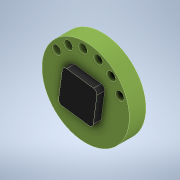
# Autodesk Inventor part: FootSensorPCB
Saved by Autodesk Inventor 2022 (Build 260153000, 153)
## iProperties
Created: 2021-12-28
Part Number: FootSensorPCB
Material: Generic
Document SubType Name: Modeling
Designer: Jochen
Density: 1 g/cm^3
Appearance: Olive Green
Author: Jochen
Autodesk Inventor part; units mm, degrees
ref_plane "YZ Plane" through (0, 0, 0) normal (1, 0, 0) x (0, 1, 0)
ref_plane "XZ Plane" through (0, 0, 0) normal (0, 1, 0) x (-1, 0, 0)
ref_plane "XY Plane" through (0, 0, 0) normal (0, 0, 1) x (1, 0, 0)
sketch "Sketch1" plane through (0, 0, 0) normal (0, 0, 1) x (1, 0, 0)
  line L0 (0, -7) -> (0, 7) construction
  line L1 (-7, 0) -> (7, 0) construction
  circle A0 centre (0, 0) radius 5
  circle A1 centre (0, 0) radius 4.2 construction
  circle A2 centre (3.8833, 1.5999) radius 0.5
  circle A3 centre (2.8968, 3.0411) radius 0.5
  circle A4 centre (1.4095, 3.9564) radius 0.5
  circle A5 centre (-0.3216, 4.1877) radius 0.5
  circle A6 centre (-1.9971, 3.6948) radius 0.5
  circle A7 centre (-3.3273, 2.5631) radius 0.5
  line L2 (1.2791, -2.1886) -> (-1.8087, -1.7762)
  line L3 (-2.1886, -1.2791) -> (-1.7762, 1.8087)
  line L4 (-1.2791, 2.1886) -> (1.8087, 1.7762)
  line L5 (2.1886, 1.2791) -> (1.7762, -1.8087)
  arc A8 (1.2791, -2.1886) -> (1.7762, -1.8087) centre (1.3377, -1.7502) ccw
  arc A9 (-2.1886, -1.2791) -> (-1.8087, -1.7762) centre (-1.7502, -1.3377) ccw
  arc A10 (-1.2791, 2.1886) -> (-1.7762, 1.8087) centre (-1.3377, 1.7502) ccw
  arc A11 (2.1886, 1.2791) -> (1.8087, 1.7762) centre (1.7502, 1.3377) ccw
  line L6 (2.8968, 3.0411) -> (-1.9971, 3.6948) construction
  line L7 (0.2648, 1.9824) -> (-0.2648, -1.9824) construction
  dimension "d1" = 8.4
  dimension "d0" = 10
  dimension "d2" = 1
  dimension "d5" = 120
  dimension "d9" = 4
  constraints: 12 end point, 11 centre point, 8 point on circle, 8 tangent, 4 midpoint, 3 coincident, 3 equal radius, 3 parallel, 3 perpendicular, 14 other
  measures "d0" diameter of A0
  measures "d2" diameter of A2
  measures "d9" distance between parallel lines of L2 L4
extrude "Extrusion1" add sketch "Sketch1" along normal blind 1.9 contours A0 | L2 A9 L3 A10 L4 A11 L5 A8
extrude "Extrusion2" add sketch "Sketch1" along normal blind 0.9 from surface at 1.9 contours L2 A9 L3 A10 L4 A11 L5 A8
body "Solid1"
